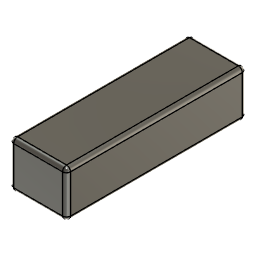
assembly_chassis (Autodesk Fusion 360 archive; units mm, degrees)
design "Batterie"
Autodesk Fusion 360 part; units mm, degrees
sketch "Skizze1" plane through (0, 0, 0) normal (0, 0, 1) x (1, 0, 0)
  line L0 (0, 0) -> (-43, 0)
  line L1 (-43, 0) -> (-43, 136)
  line L2 (-43, 136) -> (0, 136)
  line L3 (0, 136) -> (0, 0)
  dimension "d1" = 43
  dimension "d2" = 136
  constraint horizontal L0
  constraint vertical L1
  constraint horizontal L2
  constraint vertical L3
  constraint coincident L0.start L3.end
  measures "d1" distance of L0.start L0.end
  measures "d2" distance of L0.start L2.end
extrude "Extrusion1" add sketch "Skizze1" along normal blind 35
fillet "Abrundung1" radius 3 12 edges at (0, 68, 35) (-21.5, 0, 35) (-43, 68, 35) (-21.5, 136, 35) (0, 68, 0) (-21.5, 0, 0) (0, 0, 17.5) (-43, 0, 17.5) (0, 136, 17.5) (-43, 136, 17.5) (-21.5, 136, 0) (-43, 68, 0)
